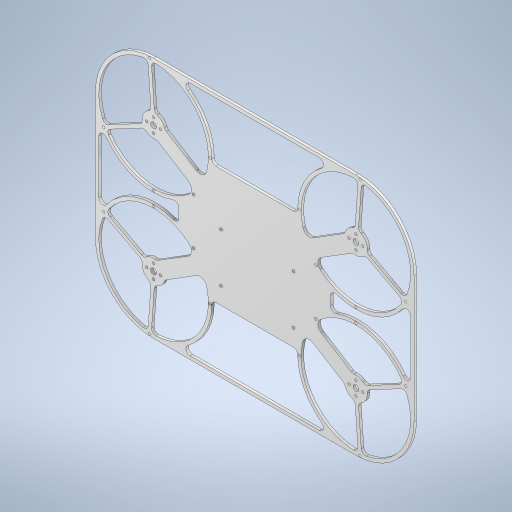
# Autodesk Inventor part: v3_bottom_carbon_fiber_new
Saved by Autodesk Inventor 2024 (Build 280153000, 153)
## iProperties
Created: 2025-03-06
Part Number: v3_bottom_carbon_fiber_new
Material: Generic
Document SubType Name: Modeling
Designer: Bruno
Density: 1 g/cm^3
Appearance: Default
Author: Bruno
Autodesk Inventor part; units mm, degrees
ref_plane "YZ Plane" through (0, 0, 0) normal (1, 0, 0) x (0, 1, 0)
ref_plane "XZ Plane" through (0, 0, 0) normal (0, 1, 0) x (-1, 0, 0)
ref_plane "XY Plane" through (0, 0, 0) normal (0, 0, 1) x (1, 0, 0)
sketch "Sketch1" plane through (0, 0, 0) normal (0, 0, 1) x (1, 0, 0)
  circle A0 centre (120, 75) radius 65
  circle A1 centre (120, 75) radius 69
  line L0 (-120, 75) -> (120, 75)
  line L1 (-120, 75) -> (-120, -75)
  line L2 (-120, -75) -> (120, -75)
  line L3 (120, -75) -> (120, 75)
  line L4 (-236.9943, 0) -> (244.4628, 0)
  line L5 (0, 171.5298) -> (0, -171.5298)
  line L6 (51.1814, 70) -> (0, 70)
  line L7 (90, 12.8631) -> (90, 0)
  line L8 (189, 75) -> (189, 0)
  line L9 (120, 144) -> (0, 144)
  circle A2 centre (120, -75) radius 65
  circle A3 centre (120, -75) radius 69
  line L10 (51.1814, -70) -> (0, -70)
  line L11 (90, -12.8631) -> (90, 0)
  line L12 (189, -75) -> (189, 0)
  line L13 (120, -144) -> (0, -144)
  line L14 (120, 140) -> (0, 140)
  line L15 (185, 75) -> (185, 0)
  line L16 (120, -140) -> (0, -140)
  line L17 (185, -75) -> (185, 0)
  circle A4 centre (-120, 75) radius 65
  circle A5 centre (-120, 75) radius 69
  line L18 (-51.1814, 70) -> (0, 70)
  line L19 (-90, 12.8631) -> (-90, 0)
  line L20 (-189, 75) -> (-189, 0)
  line L21 (-120, 144) -> (0, 144)
  line L22 (-120, -144) -> (0, -144)
  circle A6 centre (-120, -75) radius 69
  circle A7 centre (-120, -75) radius 65
  line L23 (-51.1814, -70) -> (0, -70)
  line L24 (-189, -75) -> (-189, 0)
  line L25 (-90, -12.8631) -> (-90, 0)
  line L26 (-120, 140) -> (0, 140)
  line L27 (-185, 75) -> (-185, 0)
  line L28 (-120, -140) -> (0, -140)
  line L29 (-185, -75) -> (-185, 0)
  circle A8 centre (124.8837, 141.8218) radius 1.5
  circle A9 centre (179.1604, 43.551) radius 1.5
  circle A10 centre (120, 8) radius 1.5
  circle A11 centre (53, 75) radius 1.5
  circle A12 centre (72.6238, 27.6238) radius 1.5
  circle A13 centre (124.8837, -141.8218) radius 1.5
  circle A14 centre (179.1604, -43.551) radius 1.5
  circle A15 centre (120, -8) radius 1.5
  circle A16 centre (53, -75) radius 1.5
  circle A17 centre (72.6238, -27.6238) radius 1.5
  circle A18 centre (-124.8837, 141.8218) radius 1.5
  circle A19 centre (-179.1604, 43.551) radius 1.5
  circle A20 centre (-120, 8) radius 1.5
  circle A21 centre (-53, 75) radius 1.5
  circle A22 centre (-72.6238, 27.6238) radius 1.5
  circle A23 centre (-124.8837, -141.8218) radius 1.5
  circle A24 centre (-53, -75) radius 1.5
  circle A25 centre (-72.6238, -27.6238) radius 1.5
  circle A26 centre (-120, -8) radius 1.5
  circle A27 centre (-179.1604, -43.551) radius 1.5
  line L30 (-120, -75) -> (120, 75)
  line L31 (72.6238, 27.6238) -> (120, 75)
  line L32 (124.8837, 141.8218) -> (120, 75)
  line L33 (120, 75) -> (179.1604, 43.551)
  circle A28 centre (120, 75) radius 67
  circle A29 centre (120, 75) radius 13.5
  circle A30 centre (120, 75) radius 3.5
  circle A31 centre (111.8685, 75) radius 1.5
  circle A32 centre (120, 75) radius 8.1315
  circle A33 centre (120, 66.8685) radius 1.5
  circle A34 centre (128.1315, 75) radius 1.5
  circle A35 centre (120, 83.1315) radius 1.5
  line L34 (116.2372, 62.035) -> (70.181, 33.2499)
  line L35 (106.6972, 77.299) -> (60.641, 48.5139)
  line L36 (122.9679, 88.1697) -> (126.7304, 139.6506)
  line L37 (130.8501, 66.9672) -> (176.4285, 42.7382)
  line L38 (118.9785, 88.4613) -> (122.741, 139.9422)
  line L39 (132.7276, 70.4992) -> (178.3061, 46.2702)
  circle A36 centre (120, -75) radius 13.5
  circle A37 centre (120, -75) radius 3.5
  circle A38 centre (111.8685, -75) radius 1.5
  circle A39 centre (120, -66.8685) radius 1.5
  circle A40 centre (128.1315, -75) radius 1.5
  circle A41 centre (120, -83.1315) radius 1.5
  line L40 (116.2372, -62.035) -> (70.181, -33.2499)
  line L41 (106.6972, -77.299) -> (60.641, -48.5139)
  line L42 (122.9679, -88.1697) -> (126.7304, -139.6506)
  line L43 (130.8501, -66.9672) -> (176.4285, -42.7382)
  line L44 (118.9785, -88.4613) -> (122.741, -139.9422)
  line L45 (132.7276, -70.4992) -> (178.3061, -46.2702)
  circle A42 centre (-120, 75) radius 13.5
  circle A43 centre (-120, 75) radius 3.5
  circle A44 centre (-111.8685, 75) radius 1.5
  circle A45 centre (-120, 66.8685) radius 1.5
  circle A46 centre (-128.1315, 75) radius 1.5
  circle A47 centre (-120, 83.1315) radius 1.5
  line L46 (-116.2372, 62.035) -> (-70.181, 33.2499)
  line L47 (-106.6972, 77.299) -> (-60.641, 48.5139)
  line L48 (-122.9679, 88.1697) -> (-126.7304, 139.6506)
  line L49 (-130.8501, 66.9672) -> (-176.4285, 42.7382)
  line L50 (-118.9785, 88.4613) -> (-122.741, 139.9422)
  line L51 (-132.7276, 70.4992) -> (-178.3061, 46.2702)
  circle A48 centre (-120, -75) radius 13.5
  circle A49 centre (-120, -75) radius 3.5
  line L52 (-132.7276, -70.4992) -> (-178.3061, -46.2702)
  line L53 (-130.8501, -66.9672) -> (-176.4285, -42.7382)
  line L54 (-116.2372, -62.035) -> (-70.181, -33.2499)
  line L55 (-106.6972, -77.299) -> (-60.641, -48.5139)
  line L56 (-118.9785, -88.4613) -> (-122.741, -139.9422)
  line L57 (-122.9679, -88.1697) -> (-126.7304, -139.6506)
  circle A50 centre (-120, -66.8685) radius 1.5
  circle A51 centre (-128.1315, -75) radius 1.5
  circle A52 centre (-120, -83.1315) radius 1.5
  circle A53 centre (-111.8685, -75) radius 1.5
  point P0 (0, 0)
  point P1 (-120, 0)
  point P2 (120, 0)
  point P3 (0, 75)
  point P4 (-96.8483, 140)
  point P5 (96.8483, 140)
  point P6 (96.8483, -140)
  point P7 (-96.8483, -140)
  point P8 (-185, -51.8483)
  point P9 (-185, 51.8483)
  point P10 (185, -51.8483)
  point P11 (185, 51.8483)
  point P12 (0, 0)
  point P13 (106.6972, 77.299)
  point P14 (60.641, 48.5139)
  point P15 (178.3061, 46.2702)
  point P16 (122.741, 139.9422)
  point P17 (118.9785, 88.4613)
  dimension "d71" = 16.263
  dimension "d2" = 240
  dimension "d3" = 150
  dimension "d7" = 138
  dimension "d16" = 140
  dimension "d17" = 180
  dimension "d18" = 4
  dimension "d19" = 4
  dimension "d35" = 3
  dimension "d36" = 3
  dimension "d37" = 3
  dimension "d40" = 3
  dimension "d42" = 3
  dimension "d62" = 45
  dimension "d63" = 130
  dimension "d64" = 120
  dimension "d65" = 126.185
  dimension "d66" = 134
  dimension "d67" = 27
  dimension "d68" = 7
  dimension "d69" = 3
  dimension "d74" = 360
  dimension "d76" = 18
  dimension "d77" = 4
  dimension "d78" = 4
  constraints: 116 end point, 105 symmetric about line, 53 centre point, 40 point on circle, 13 coincident, 12 point on line, 7 perpendicular, 4 midpoint, 3 horizontal, 3 parallel, 2 tangent, 1 horizontal alignment, 1 vertical, 50 other
  measures "d2" distance of L0.start L0.end
  measures "d3" distance of L2.end L0.end
  measures "d7" diameter of A1
  measures "d16" diameter of L6 L4
  measures "d17" diameter of L7 L5
  measures "d18" distance between parallel lines of L9 L14
  measures "d19" distance between parallel lines of L8 L15
  measures "d35" diameter of A8
  measures "d36" diameter of A9
  measures "d37" diameter of A10
  measures "d40" diameter of A11
  measures "d42" diameter of A12
  measures "d62" angle of L0 L31
  measures "d63" diameter of A0
  measures "d64" angle of L30 L33
  measures "d65" angle of L30 L32
  measures "d66" diameter of A28
  measures "d67" diameter of A29
  measures "d68" diameter of A30
  measures "d69" diameter of A31
  measures "d76" diameter of L34 L30
  measures "d77" diameter of L36 L32
  measures "d78" diameter of L37 L33
extrude "Extrusion1" add sketch "Sketch1" along normal blind 3 contours L15 A28 A9 L33 A0 | A0 L32 A8 A28 L15 | L36 A29 L32 A0 | A0 L33 A29 L39 | A28 A8 L14 A1 L15 | L15 A1 L3 A10 A28 A9 | L32 A29 L38 A0 | A0 L14 A28 A8 L32 | A29 L33 A32 A34 A35 L32 | L33 A9 A28 A10 L3 A0 | A0 L37 A29 L33 | A1 L8 L4 L15 | L32 A35 A32 A31 L0 A29 | A29 L3 A33 A32 L33 | A1 L30 A28 A12 A10 L3 | L4 L12 A3 L17 | A0 L0 A11 A28 L14 | L3 A10 A28 A12 L31 A0 | A32 A33 L3 A30 L33 | L33 A30 L32 A35 A32 A34 | L7 L4 L30 A1 | A1 L14 L5 L9 | L17 A2 L3 A15 A3 | A3 L16 A2 L17 | A0 L30 A28 A11 L0 | A28 A11 L0 A1 L14 | A29 L0 L35 | A35 L32 A30 L0 A31 A32 | L31 A12 A28 L30 A0 | A29 L31 A32 A33 L3 | L30 L5 L6 A1 | A1 L0 A11 A28 L30 | L11 A3 L10 L5 L4 | L3 A15 A2 L2 A16 A3 | L5 L26 A5 L21 | L35 L0 A29 L30 A0 | L0 A31 A32 L30 A29 | A0 L30 A29 L31 L34 | L31 A29 L34 | L3 A33 A32 L31 A30 | L30 A6 L25 L4 | L4 L19 A5 L18 L5 | L5 L23 A6 L30 | A5 L26 A4 L27 | L13 L5 L16 A3 | L45 A36 L43 A2 | A2 L44 A36 L42 | L30 A32 L31 A29 | L0 A30 L30 A32 A31 | A30 L31 A32 L30 | L30 A7 L1 A26 A6 | A6 L2 A24 A7 L30 | A5 L0 A21 A4 L26 | A5 L27 L4 L20 | A3 L2 A16 A2 L16 | L22 A6 L28 L5 | A36 L2 A38 A37 L3 A39 | A5 L1 A20 A4 L0 A21 | L30 A48 L54 A7 | A7 L55 L2 A48 L30 | L27 A4 L1 A20 A5 | L4 L29 A6 L24 | A6 L29 A7 L28 | L1 A26 A7 L29 A6 | A6 L28 A7 L2 A24 | A48 L2 A53 A49 L30 | L30 A49 L1 A50 A48 | L3 A39 A37 L2 A38 A36 | L40 A36 L2 L41 A2 | L50 A42 L48 A4 | L41 L2 A36 | L55 A48 L2 | A48 L1 A50 A49 L2 A53 | L47 A4 L46 A42 L0 | L0 A42 L47 | A42 L0 A44 A43 L1 A45 | L51 A42 L49 A4 | L53 A48 L52 A7 | A42 L1 A45 A43 L0 A44 | A7 L57 A48 L56
fillet "Fillet1" radius 5 48 edges at (-185, 51.8483, 1.5) (-185, -51.8483, 1.5) (-90, 12.8631, 1.5) (-90, -12.8631, 1.5) (-51.1814, 70, 1.5) (51.1814, 70, 1.5) (96.8483, 140, 1.5) (-96.8483, 140, 1.5) (90, 12.8631, 1.5) (90, -12.8631, 1.5) (51.1814, -70, 1.5) (-51.1814, -70, 1.5) (-96.8483, -140, 1.5) (185, 51.8483, 1.5) (185, -51.8483, 1.5) (96.8483, -140, 1.5) (-130.8501, 66.9672, 1.5) (-118.9785, 88.4613, 1.5) (-122.9679, 88.1697, 1.5) (-132.7276, 70.4992, 1.5) (-126.7304, 139.6506, 1.5) (-122.741, 139.9422, 1.5) (-176.4285, 42.7382, 1.5) (-178.3061, 46.2702, 1.5) (-178.3061, -46.2702, 1.5) (-176.4285, -42.7382, 1.5) (-132.7276, -70.4992, 1.5) (-130.8501, -66.9672, 1.5) (-122.9679, -88.1697, 1.5) (-118.9785, -88.4613, 1.5) (-126.7304, -139.6506, 1.5) (-122.741, -139.9422, 1.5) (122.741, -139.9422, 1.5) (126.7304, -139.6506, 1.5) (122.9679, -88.1697, 1.5) (118.9785, -88.4613, 1.5) (132.7276, -70.4992, 1.5) (130.8501, -66.9672, 1.5) (178.3061, -46.2702, 1.5) (176.4285, -42.7382, 1.5) (178.3061, 46.2702, 1.5) (176.4285, 42.7382, 1.5) (126.7304, 139.6506, 1.5) (122.741, 139.9422, 1.5) (132.7276, 70.4992, 1.5) (130.8501, 66.9672, 1.5) (122.9679, 88.1697, 1.5) (118.9785, 88.4613, 1.5)
fillet "Fillet2" radius 5 8 edges at (116.2372, 62.035, 1.5) (106.6972, 77.299, 1.5) (116.2372, -62.035, 1.5) (106.6972, -77.299, 1.5) (-106.6972, -77.299, 1.5) (-116.2372, -62.035, 1.5) (-106.6972, 77.299, 1.5) (-116.2372, 62.035, 1.5)
fillet "Fillet3" radius 8 8 edges at (-60.641, -48.5139, 1.5) (-70.181, -33.2499, 1.5) (-70.181, 33.2499, 1.5) (-60.641, 48.5139, 1.5) (70.181, 33.2499, 1.5) (60.641, 48.5139, 1.5) (70.181, -33.2499, 1.5) (60.641, -48.5139, 1.5)
sketch "Sketch2" plane through (0, 0, 3) normal (0, 0, 1) x (1, 0, 0)
  line L0 (-257.4929, 0) -> (257.4929, 0)
  line L1 (0, 204.3201) -> (0, -204.3201)
  line L2 (-40, -50) -> (46, -50)
  line L3 (46, -50) -> (46, 8)
  line L4 (46, 8) -> (-40, 8)
  line L5 (-40, 8) -> (-40, -50)
  circle A0 centre (-40, -50) radius 1.5
  circle A1 centre (46, -50) radius 1.5
  circle A2 centre (46, 8) radius 1.5
  circle A3 centre (-40, 8) radius 1.5
  line L6 (-46, -70) -> (46, -70) projected
  point P0 (0, 0)
  point P1 (0, 0)
  dimension "d45" = 86
  dimension "d46" = 58
  dimension "d47" = 3
  dimension "d48" = 3
  dimension "d49" = 3
  dimension "d50" = 3
  dimension "d52" = 40
  dimension "d55" = 20
  constraints: 12 end point, 5 coincident, 4 centre point, 2 horizontal, 2 midpoint, 2 parallel, 1 perpendicular, 1 vertical
  measures "d45" distance of L2.start L2.end
  measures "d46" distance of L4.end L2.start
  measures "d47" diameter of A3
  measures "d48" diameter of A0
  measures "d49" diameter of A1
  measures "d50" diameter of A2
  measures "d52" distance between parallel lines of L5 L1
  measures "d55" distance between parallel lines of L6 L2
extrude "Extrusion2" cut sketch "Sketch2" against normal through all contours A3 L4 L5 | L5 L4 A3 | A0 L2 L5 | L5 L2 A0 | A1 L2 L3 | L3 L2 A1 | A2 L4 L3 | L3 L4 A2
sketch "Sketch3" plane through (0, 0, 0) normal (0, 0, -1) x (-1, 0, 0)
  line L0 (122.5, -100) -> (-122.5, -100)
  line L1 (-122.5, -100) -> (-122.5, 100)
  line L2 (-122.5, 100) -> (122.5, 100)
  line L3 (122.5, 100) -> (122.5, -100)
  line L4 (122.5, -100) -> (-122.5, 100)
  line L5 (202.5, -160) -> (-202.5, -160)
  line L6 (-202.5, -160) -> (-202.5, 160)
  line L7 (-202.5, 160) -> (202.5, 160)
  line L8 (202.5, 160) -> (202.5, -160)
  line L9 (-202.5, -160) -> (202.5, 160)
  point P0 (0, 0)
  point P1 (0, 0)
  dimension "d56" = 200
  dimension "d57" = 245
  dimension "d58" = 60
  dimension "d59" = 80
  constraints: 20 end point, 4 parallel, 2 horizontal, 2 midpoint, 2 perpendicular, 1 coincident
  measures "d56" distance of L2.end L0.start
  measures "d57" distance of L0.start L0.end
  measures "d58" distance between parallel lines of L0 L5
  measures "d59" distance between parallel lines of L8 L3
body "Solid1"
